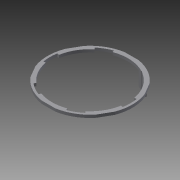
# Autodesk Inventor part: nose
Saved by Autodesk Inventor 2015 (Build 190159000, 159)
## iProperties
Created: 2019-10-01
Part Number: nose
Material: Generic
Document SubType Name: Modeling
Designer: gabri
Density: 1 g/cm^3
Appearance: Default
Author: gabri
Autodesk Inventor part; units mm, degrees
ref_plane "YZ Plane" through (0, 0, 0) normal (1, 0, 0) x (0, 1, 0)
ref_plane "XZ Plane" through (0, 0, 0) normal (0, 1, 0) x (-1, 0, 0)
ref_plane "XY Plane" through (0, 0, 0) normal (0, 0, 1) x (1, 0, 0)
sketch "Sketch1" plane through (0, 0, 0) normal (0, 0, 1) x (1, 0, 0)
  line L0 (-17.4274, 20.6224) -> (-18.3956, 21.7681) projected
  arc A0 (-9.8513, 26.7432) -> (-18.3956, 21.7681) centre (0, 0) ccw projected
  line L1 (-9.8513, 26.7432) -> (-9.3328, 25.3357) projected
  arc A1 (9.1458, 25.4038) -> (-9.3328, 25.3357) centre (0, 0) ccw projected
  line L2 (9.1458, 25.4038) -> (9.6539, 26.8151) projected
  arc A2 (18.2347, 21.9031) -> (9.6539, 26.8151) centre (0, 0) ccw projected
  line L3 (18.2347, 21.9031) -> (17.2749, 20.7503) projected
  arc A3 (26.5733, 4.7814) -> (17.2749, 20.7503) centre (0, 0) ccw projected
  line L4 (26.5733, 4.7814) -> (28.0496, 5.047) projected
  arc A4 (28.086, -4.8401) -> (28.0496, 5.047) centre (0, 0) ccw projected
  line L5 (28.086, -4.8401) -> (26.6078, -4.5854) projected
  arc A5 (17.4274, -20.6224) -> (26.6078, -4.5854) centre (0, 0) ccw projected
  line L6 (17.4274, -20.6224) -> (18.3956, -21.7681) projected
  arc A6 (9.8513, -26.7432) -> (18.3956, -21.7681) centre (0, 0) ccw projected
  line L7 (9.8513, -26.7432) -> (9.3328, -25.3357) projected
  arc A7 (-9.1458, -25.4038) -> (9.3328, -25.3357) centre (0, 0) ccw projected
  line L8 (-9.1458, -25.4038) -> (-9.6539, -26.8151) projected
  arc A8 (-18.2347, -21.9031) -> (-9.6539, -26.8151) centre (0, 0) ccw projected
  line L9 (-18.2347, -21.9031) -> (-17.2749, -20.7503) projected
  arc A9 (-26.5733, -4.7814) -> (-17.2749, -20.7503) centre (0, 0) ccw projected
  line L10 (-26.5733, -4.7814) -> (-28.0496, -5.047) projected
  arc A10 (-28.086, 4.8401) -> (-28.0496, -5.047) centre (0, 0) ccw projected
  line L11 (-28.086, 4.8401) -> (-26.6078, 4.5854) projected
  arc A11 (-17.4274, 20.6224) -> (-26.6078, 4.5854) centre (0, 0) ccw projected
  arc A12 (-4.9259, 29.5928) -> (-23.3051, 18.8911) centre (0, 0) ccw projected
  line L12 (-23.3051, 18.8911) -> (-28.0911, 10.5304) projected
  arc A13 (-28.0911, 10.5304) -> (-28.0127, -10.7372) centre (0, 0) ccw projected
  line L13 (-28.0127, -10.7372) -> (-23.1652, -19.0624) projected
  arc A14 (-23.1652, -19.0624) -> (-4.7077, -29.6283) centre (0, 0) ccw projected
  line L14 (-4.7077, -29.6283) -> (4.9259, -29.5928) projected
  arc A15 (4.9259, -29.5928) -> (23.3051, -18.8911) centre (0, 0) ccw projected
  line L15 (23.3051, -18.8911) -> (28.0911, -10.5304) projected
  arc A16 (28.0911, -10.5304) -> (28.0127, 10.7372) centre (0, 0) ccw projected
  line L16 (28.0127, 10.7372) -> (23.1652, 19.0624) projected
  arc A17 (23.1652, 19.0624) -> (4.7077, 29.6283) centre (0, 0) ccw projected
  line L17 (4.7077, 29.6283) -> (-4.9259, 29.5928) projected
  point P0 (0, 0)
extrude "Extrusion1" add sketch "Sketch1" along normal blind 2
sketch "Sketch2" plane through (0, 0, 2) normal (0, 0, 1) x (1, 0, 0)
  line L0 (12.6834, 23.9683) -> (12.6247, 23.8666) projected
  line L1 (14.4155, 22.9683) -> (12.6834, 23.9683) projected
  line L2 (14.3568, 22.8666) -> (14.4155, 22.9683) projected
  arc A0 (17.2749, 20.7503) -> (14.3568, 22.8666) centre (0, 0) ccw projected
  line L3 (18.2347, 21.9031) -> (17.2749, 20.7503) projected
  arc A1 (18.2347, 21.9031) -> (9.6539, 26.8151) centre (0, 0) ccw projected
  line L4 (9.1458, 25.4038) -> (9.6539, 26.8151) projected
  arc A2 (12.6247, 23.8666) -> (9.1458, 25.4038) centre (0, 0) ccw projected
  point P0 (0, 0)
extrude "Extrusion2" add sketch "Sketch2" against normal blind 12
sketch "Sketch3" plane through (12.6834, 23.9683, -10) normal (-0.5, -0.8660254, 0) x (0.8660254, -0.5, 0)
  spline S0 degree 3 poles (0.1034, 6) (0.1034, 6.1256) (0.1285, 6.2595) (0.2306, 6.5059) (0.3076, 6.6183) (0.4851, 6.7959) (0.5976, 6.8729) (0.8439, 6.9749) (0.9779, 7) (1.229, 7) (1.363, 6.9749) (1.6093, 6.8728) (1.7218, 6.7959) (1.8993, 6.6183) (1.9763, 6.5059) (2.0783, 6.2595) (2.1034, 6.1256) (2.1034, 5.8744) (2.0783, 5.7405) (1.9763, 5.4941) (1.8993, 5.3817) (1.7218, 5.2041) (1.6093, 5.1272) (1.363, 5.0251) (1.229, 5) (0.9779, 5) (0.8439, 5.0251) (0.5976, 5.1271) (0.4851, 5.2041) (0.3076, 5.3817) (0.2306, 5.4941) (0.1285, 5.7405) (0.1034, 5.8744) (0.1034, 6) knots 0 0 0 0 0.037671 0.037671 0.075343 0.075343 0.113013 0.113013 0.150683 0.150683 0.188357 0.188357 0.226031 0.226031 0.263702 0.263702 0.301374 0.301374 0.339046 0.339046 0.376718 0.376718 0.414391 0.414391 0.452065 0.452065 0.489735 0.489735 0.527405 0.527405 0.565077 0.565077 0.602748 0.602748 0.602748 0.602748 projected
  point P0 (1, 10)
  point P1 (0.1034, 6)
  point P2 (1, 6)
hole "Hole1" at (13.5495, 23.4683, -4) direction (0.5, 0.8660254, 0) diameter 1.5 depth 8 tip angle 118
pattern_circular "Circular Pattern1" count 6 over 360 about axis through (0, 0, 0) along (0, 0, 1) of "Hole1", "Extrusion2"
sketch "Sketch4" plane through (0, 0, 2) normal (0, 0, 1) x (1, 0, 0)
  arc A0 (-4.9259, 29.5928) -> (-23.3051, 18.8911) centre (0, 0) ccw projected
  arc A1 (-4.9259, 29.5928) -> (-23.3051, 18.8911) centre (0, 0) ccw projected
  point P0 (0, 0)
ref_plane "Work Plane1" through (-2.3928, -4.1804, 0) normal (-0.8678623, 0.4968048, 0) x (0, 0, 1)
sketch "Sketch5" plane through (-2.3928, -4.1804, 0) normal (-0.8678623, 0.4968048, 0) x (0, 0, 1)
  line L0 (2, 32.8689) -> (2, 34.8168) projected
  line L1 (2, 34.8168) -> (4.0385, 34.8168)
  line L2 (2, 33.3168) -> (4.1605, 33.3168)
  line L3 (0, 4.8168) -> (20, 4.8168)
  line L4 (0, 0) -> (0, 9.6336) projected
  ellipse E0 centre (4.1605, 4.8168) end of major axis (3.8849, 34.8168) minor radius 15.839 (10, 32.5634) -> (2, 34.5858) ccw
  line L5 (9.4222, 30.9602) -> (10, 32.5634)
  ellipse E1 centre (4.1605, 4.8168) end of major axis (3.8987, 33.3165) minor radius 13.6786 (9.4222, 30.9602) -> (3.959, 33.3168) ccw
  dimension "d15" = 1.5
  dimension "d16" = 20
  constraints: 8 end point, 4 point on line, 3 horizontal, 1 perpendicular, 9 other
  measures "d15" distance between parallel lines of L1 L2
  measures "d16" distance of L3.start L3.end
revolve "Revolution1" add sketch "Sketch5" angle 360 about axis through (0.0002, -0.0001, 0) along (0, 0, 1)
sketch "Sketch6" plane through (-2.3928, -4.1804, 0) normal (-0.8678623, 0.4968048, 0) x (0, 0, 1)
  line L0 (0, 4.8168) -> (-5, 4.8168)
  ellipse E0 centre (-4, 31.9155) end of major axis (-4.75, 31.9155) minor radius 0.0028 projected
  line L1 (2, 31.9119) -> (2, 31.9192) projected
  line L2 (2, 31.9192) -> (-10, 31.9192) projected
  line L3 (-10, 31.9119) -> (-10, 31.9192) projected
  line L4 (2, 31.9119) -> (-10, 31.9119) projected
  line L5 (2, 31.9192) -> (2, 28.9192)
  line L6 (2, 31.7944) -> (2, 19.0892) projected
  line L7 (0, 31.9119) -> (0, 29.9748)
  line L8 (-5, 4.8168) -> (-5, 13.1213)
  line L9 (-5, 13.1213) -> (2, 28.9192)
  line L10 (0, 31.9192) -> (0, 29.3425)
  line L11 (0, 29.3425) -> (-7, 13.5445)
  line L12 (-7, 13.5445) -> (-7, 4.8168)
  line L13 (-5, 4.8168) -> (-7, 4.8168)
  line L14 (0, 31.9192) -> (2, 31.9192)
  dimension "d18" = 5
  dimension "d19" = 3
  dimension "d20" = 2
  constraints: 20 end point, 2 point on line, 2 vertical, 1 collinear, 1 horizontal, 1 perpendicular, 2 other
  measures "d18" distance of L0.start L0.end
  measures "d19" distance of L1.end L5.end
  measures "d20" distance between parallel lines of L8 L12
revolve "Revolution2" add sketch "Sketch6" angle 360 about axis through (0.0002, -0.0001, 0) along (0, 0, -1) contours L10 L2 L1 L4 | L4 L5 L9 L8 L13 L12 L11 L10 L7
sketch "Sketch8" plane through (0.0002, -0.0001, -7) normal (0, 0, -1) x (-1, 0, 0)
  line L0 (0.0002, 0.0001) -> (0.0002, 10.6925)
  point P0 (0.0002, 4.0001)
  dimension "d30" = 4
  constraints: 2 end point, 1 vertical
  measures "d30" distance of L0.start point (0, 4)
hole "Hole3" at (0, 4, -7) direction (0, 0, 1) diameter 2 depth 100 tip angle 118
pattern_linear "Rectangular Pattern1" count 7 spacing 3 along (0, 1, 0) of "Hole3"
pattern_circular "Circular Pattern2" count 8 over 360 about axis through (0.0002, -0.0001, -3.5) along (0, 0, 1) of "Hole3", "Rectangular Pattern1"
sketch "Sketch9" plane through (0.0002, -0.0001, -7) normal (0, 0, -1) x (-1, 0, 0)
  circle A0 centre (-4.9497, 4.95) radius 1 projected
  circle A1 centre (0.0002, 7.0001) radius 1 projected
  line L0 (-4.9497, 4.95) -> (0.0002, 7.0001)
  line L1 (0.0002, 0.0001) -> (-2.4747, 5.975)
  constraints: 4 end point, 1 midpoint
hole "Hole4" at (2.4749, 5.9749, -7) direction (0, 0, 1) diameter 2 depth 100 tip angle 118
pattern_linear "Rectangular Pattern2" count 5 spacing 4 along (0.3826894, 0.9238771, 0) of "Hole4"
pattern_circular "Circular Pattern3" count 8 over 360 about axis through (0.0002, -0.0001, -3.5) along (0, 0, 1) of "Hole4", "Rectangular Pattern2"
sketch "Sketch10" plane through (0.0002, -0.0001, -5) normal (0, 0, 1) x (1, 0, 0)
  circle A0 centre (-0.0002, 0.0001) radius 8.2801
  constraints: 1 centre point, 1 coincident
extrude "Extrusion3" add sketch "Sketch10" against normal blind 2
sketch "Sketch11" plane through (0.0002, -0.0001, -5) normal (0, 0, 1) x (1, 0, 0)
  point P0 (-0.0002, 0.0001)
sketch "Sketch12" plane through (0.0002, -0.0001, -5) normal (0, 0, 1) x (1, 0, 0)
  point P0 (-0.0002, 0.0001)
  point P1 (-0.0002, -15.9376)
  point P2 (-0.0002, 15.9376)
  constraints: 2 other
body "Solid1"
